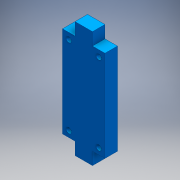
# Autodesk Inventor part: backFrame
Saved by Autodesk Inventor 2016 (Build 200138000, 138)
## iProperties
Created: 2016-06-05
Part Number: backFrame
Material: Generic
Document SubType Name: Modeling
Designer: hesaon
Density: 1 g/cm^3
Appearance: Default
Author: hesaon
Autodesk Inventor part; units mm, degrees
ref_plane "YZ Plane" through (0, 0, 0) normal (1, 0, 0) x (0, 1, 0)
ref_plane "XZ Plane" through (0, 0, 0) normal (0, 1, 0) x (-1, 0, 0)
ref_plane "XY Plane" through (0, 0, 0) normal (0, 0, 1) x (1, 0, 0)
sketch "Sketch1" plane through (0, 0, 0) normal (0, 1, 0) x (-1, 0, 0)
  line L0 (0, 0) -> (10, 0)
  line L1 (10, 0) -> (10, 10)
  line L2 (10, 10) -> (24, 10)
  line L3 (24, 10) -> (24, 0)
  line L4 (24, 0) -> (34, 0)
  line L5 (34, 0) -> (34, -73)
  line L6 (34, -73) -> (24, -73)
  line L7 (24, -73) -> (24, -83)
  line L8 (24, -83) -> (10, -83)
  line L9 (10, -83) -> (10, -73)
  line L10 (10, -73) -> (0, -73)
  line L11 (0, -73) -> (0, 0)
  dimension "d9" = 73
  dimension "d10" = 34
  dimension "thickness" = 10
  dimension "t" = 10
  dimension "d13" = 10
  dimension "d14" = 10
  dimension "d15" = 10
  dimension "d16" = 10
  dimension "d17" = 10
  constraints: 24 end point, 11 perpendicular, 1 coincident, 1 point on line, 1 vertical
  measures "d9" distance of L10.end point (0, 0)
  measures "d10" distance of point (0, 0) L4.end
  measures "thickness" distance of L0.end L1.end
  measures "t" distance of point (0, 0) L0.end
  measures "d13" distance of L3.end L4.end
  measures "d14" distance of L6.end L5.end
  measures "d15" distance of L8.end L9.end
  measures "d16" distance of L7.end L6.end
  measures "d17" distance from line of L11 L8.end
extrude "Extrusion1" add sketch "Sketch1" along normal blind 10
hole "Hole1" at (-29, 10, -5) direction (0, -1, 0) diameter 4.3 end through all
hole "Hole2" at (-5, 10, -5) direction (0, -1, 0) diameter 4.3 end through all
hole "Hole3" at (-5, 10, -68) direction (0, -1, 0) diameter 4.3 end through all
hole "Hole4" at (-29, 10, -68) direction (0, -1, 0) diameter 4.3 end through all
equation "\"thickness\" = t"
equation "\"d13\" = t"
equation "\"d14\" = t"
equation "\"d15\" = t"
equation "\"d16\" = t"
equation "\"d17\" = t"
equation "\"d18\" = t"
body "Solid1"
